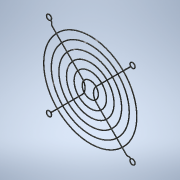
# Autodesk Inventor part: Schutzgitter
Saved by Autodesk Inventor 2021 (Build 250183000, 183)
## iProperties
Created: 2021-05-06
Part Number: Schutzgitter
Material: Stahl
Document SubType Name: Modeling
Designer: Sebastian Seewald
Density: 7.85 g/cm^3
Appearance: Platte
Mass: 8.02694 g
Surface Area: 40.9325 cm^2
Volume: 1.02254 cm^3
Author: Sebastian Seewald
Autodesk Inventor part; units mm, degrees
note: some values were not read from the file. Chosen so that the rebuilt part matches the saved one: second side of "Extrusion1".
sketch "Skizze1" plane through (0, 0, 0) normal (0, 0, 1) x (1, 0, 0)
  circle A0 centre (0, 0) radius 38.5
  circle A1 centre (0, 0) radius 23.5
  circle A2 centre (0, 0) radius 16
  circle A3 centre (0, 0) radius 8
  circle A4 centre (0, 0) radius 46
  circle A5 centre (0, 0) radius 31
  dimension "d12" = 92
  dimension "d13" = 77
  dimension "d14" = 62
  dimension "d15" = 47
  dimension "d16" = 32
  dimension "d17" = 16
  constraints: 6 centre point, 6 coincident
  measures "d12" diameter of A4
  measures "d13" diameter of A0
  measures "d14" diameter of A5
  measures "d15" diameter of A1
  measures "d16" diameter of A2
  measures "d17" diameter of A3
sketch "Skizze2" plane through (0, 0, 0) normal (0, 1, 0) x (-1, 0, 0)
  circle A0 centre (8, 0) radius 0.5
  circle A1 centre (16, 0) radius 0.5
  circle A2 centre (23.5, 0) radius 0.5
  circle A3 centre (31, 0) radius 0.5
  circle A4 centre (38.5, 0) radius 0.5
  circle A5 centre (46, 0) radius 0.5
  point P0 (0, 0)
  dimension "d20" = 1
  dimension "d21" = 8
  dimension "d22" = 1
  dimension "d23" = 16
  dimension "d24" = 1
  dimension "d25" = 23.5
  dimension "d26" = 1
  dimension "d27" = 31
  dimension "d28" = 38.5
  dimension "d29" = 1
  dimension "d30" = 1
  dimension "d31" = 46
  constraints: 6 centre point
  measures "d20" diameter of A0
  measures "d21" distance of point (0, 0) A0.centre
  measures "d22" diameter of A1
  measures "d23" distance of point (0, 0) A1.centre
  measures "d24" diameter of A2
  measures "d25" distance of point (0, 0) A2.centre
  measures "d26" diameter of A3
  measures "d27" distance of point (0, 0) A3.centre
  measures "d28" distance of point (0, 0) A4.centre
  measures "d29" diameter of A4
  measures "d30" diameter of A5
  measures "d31" distance of point (0, 0) A5.centre
sweep "Sweeping1" add profiles "Skizze2" path "Skizze1" path curves A4
ref_plane "Arbeitsebene2" through (0, 0, 1) normal (0, 0, 1) x (1, 0, 0)
sketch "Skizze3" plane through (0, 0, 1) normal (0, 0, 1) x (1, 0, 0)
  point P0 (0, 0)
sketch "Skizze4" plane through (0, 0, 1) normal (0, 0, 1) x (1, 0, 0)
  line L0 (-36, -36) -> (-7.071068, -7.071068)
  line L1 (-7.071068, 7.071068) -> (-36, 36)
  arc A0 (-7.071068, -7.071068) -> (-7.071068, 7.071068) centre (-14.142136, 0) ccw
  point P0 (0, 0)
  dimension "d35" = 36
  dimension "d36" = 36
  dimension "d37" = 36
  dimension "d38" = 36
  dimension "d39" = 10
  constraints: 4 end point, 2 point on circle, 2 point on line, 2 tangent, 1 centre point
  measures "d35" horizontal distance of point (0, 0) L0.start
  measures "d36" horizontal distance of point (0, 0) L1.end
  measures "d37" horizontal distance of point (0, 0) L0.start
  measures "d38" horizontal distance of point (0, 0) L1.end
  measures "d39" radius of A0
ref_plane "Arbeitsebene3" through (-36, -36, 1) normal (0.7071068, 0.7071068, 0) x (-0.7071068, 0.7071068, 0)
sketch "Skizze5" plane through (-36, -36, 1) normal (0.7071068, 0.7071068, 0) x (-0.7071068, 0.7071068, 0)
  circle A0 centre (0, 0) radius 0.5
  point P0 (0, -1)
  dimension "d40" = 1
  constraints: 1 centre point
  measures "d40" diameter of A0
sweep "Sweeping2" add profiles "Skizze5" path "Skizze4"
mirror "Spiegeln1" about plane through (0, 0, 0) normal (1, 0, 0) of "Sweeping2"
sketch "Skizze6" plane through (0, 0, 0) normal (0, 0, 1) x (1, 0, 0)
  circle A0 centre (-41.25, 41.25) radius 3
  circle A1 centre (-41.25, 41.25) radius 2
  point P0 (0, 0)
  dimension "d43" = 41.25
  dimension "d44" = 41.25
  dimension "d45" = 6
  dimension "d46" = 4
  constraints: 2 centre point, 1 coincident
  measures "d43" horizontal distance of point (0, 0) A0.centre
  measures "d44" horizontal distance of point (0, 0) A0.centre
  measures "d45" diameter of A0
  measures "d46" diameter of A1
extrude "Extrusion1" add sketch "Skizze6" against normal blind 1
fillet "Rundung1" radius 0.5 4 edges at (-44.25, 41.25, 0) (-44.25, 41.25, -1) (-43.25, 41.25, 0) (-43.25, 41.25, -1)
pattern_circular "Runde Anordnung1" count 4 over 360 about axis through (0, 0, -10) along (0, 0, 1) of "Extrusion1", "Rundung1"
ref_plane "Arbeitsebene4" through (-39.535534, -39.535534, 1) normal (-0.7071068, -0.7071068, 0) x (-0.7071068, 0.7071068, 0)
sketch "Skizze7" plane through (-39.535534, -39.535534, 1) normal (-0.7071068, -0.7071068, 0) x (-0.7071068, 0.7071068, 0)
  line L0 (-23.5, 1.5) -> (23.5, 1.5) projected
  circle A0 centre (0, 1.5) radius 0.5
  point P0 (0, 1)
  dimension "d56" = 1
  constraints: 1 centre point, 1 midpoint
  measures "d56" diameter of A0
ref_plane "Arbeitsebene5" through (0, 0, 0) normal (0.7071068, -0.7071068, 0) x (0, 0, 1)
sketch "Skizze8" plane through (0, 0, 0) normal (0.7071068, -0.7071068, 0) x (0, 0, 1)
  line L0 (0.5, 50.911688) -> (1.5, 50.911688)
  spline S0 degree 4 poles (-0.524018, 55.889684) (-0.524018, 54.486251) (-0.321154, 53.99791) (0.864719, 53.23055) (1.014501, 51.986577) (1, 51.308722) (1, 50.911688) knots 0 0 0 0 0 0.44074295 0.69074295 1 1 1 1 1
  line L1 (1, 51.508318) -> (1, 50.315058) construction
  arc A0 (1.00443, 51.38891) -> (1.00443, 50.434467) centre (26.703784, 50.911688) ccw construction
  line L2 (-0.524018, 57.057643) -> (-0.524018, 54.721726) construction
  arc A1 (-0.502273, 56.823037) -> (-0.502273, 54.956332) centre (19.517878, 55.889684) ccw construction
  line L3 (0.751884, 52.976787) -> (1.031828, 51.896282) construction
  arc A2 (0.964384, 52.0013) -> (0.743918, 52.852231) centre (-1.527482, 51.809715) ccw construction
  point P0 (0, 0)
  point P1 (0.163246, 53.635575)
  point P2 (0.891856, 52.436534)
  dimension "d60" = 0
  dimension "d61" = 0.5
  constraints: 6 end point, 6 midpoint, 4 vertical, 3 centre point, 3 point on circle, 8 other
  measures "d60" distance from line of L0 point (1, 50.912)
  measures "d61" distance of L0.end point (1, 50.912)
sweep "Sweeping3" add profiles "Skizze7" path "Skizze8" path curves S0
pattern_circular "Runde Anordnung2" count 4 over 360 about axis through (0, 0, -10) along (0, 0, 1) of "Sweeping3"
